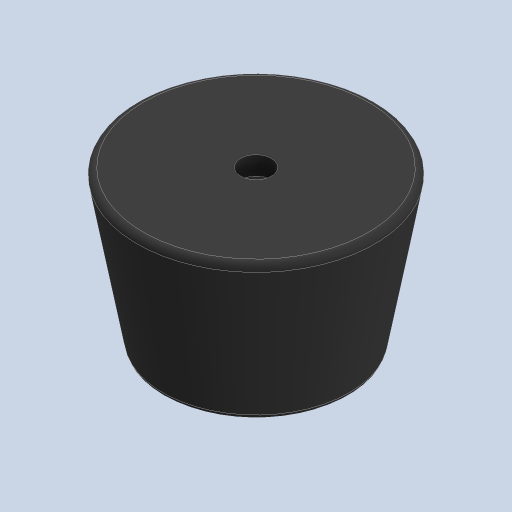
# Autodesk Inventor part: Pés
Saved by Autodesk Inventor 2023 (Build 270158000, 158)
## iProperties
Created: 2023-04-29
Part Number: Pés
Material: Rubber, Silicone
Document SubType Name: Sheet Metal
Designer: Mateus PC
Density: 1.25 g/cm^3
Sheet Metal Rule: Default_mm
Appearance: Rubber - Black
Mass: 12.8254 g
Surface Area: 66.7725 cm^2
Volume: 10.2603 cm^3
Author: Mateus PC
Autodesk Inventor part; units mm, degrees
ref_plane "YZ Plane" through (0, 0, 0) normal (1, 0, 0) x (0, 1, 0)
ref_plane "XZ Plane" through (0, 0, 0) normal (0, 1, 0) x (-1, 0, 0)
ref_plane "XY Plane" through (0, 0, 0) normal (0, 0, 1) x (1, 0, 0)
sketch "Sketch5" plane through (0, 0, 0) normal (0, 0, 1) x (1, 0, 0)
  line L0 (20, 0) -> (-20, 0) projected
  line L1 (-15.1481, 0.8228) -> (-19.2881, 23.8228)
  line L2 (-18.3039, 25) -> (-2.5, 25)
  line L3 (-2.5, 25) -> (-2.5, 22)
  line L4 (-2.5, 22) -> (-14.3283, 22)
  line L5 (-15.3159, 20.8429) -> (-12.1841, 1.1571)
  line L6 (-14.5, 0) -> (14.5, 0) projected
  arc A0 (-14.3283, 22) -> (-15.3159, 20.8429) centre (-14.3283, 21) ccw
  arc A1 (-18.3039, 25) -> (-19.2881, 23.8228) centre (-18.3039, 24) ccw
  line L7 (-14.1639, 0) -> (-13.1717, 0)
  arc A2 (-13.1717, 0) -> (-12.1841, 1.1571) centre (-13.1717, 1) ccw
  arc A3 (-15.1481, 0.8228) -> (-14.1639, 0) centre (-14.1639, 1) ccw
  line L8 (-28, 0) -> (28, 0) projected
  line L9 (0, -5.3193) -> (0, 30.3215) projected
  point P0 (0, 0)
  point P1 (-15, 0)
  point P2 (-19.5, 25)
  point P3 (-15.5, 22)
  point P4 (-12, 0)
  point P5 (0, 0)
  point P6 (0, 0)
  point P7 (-2.5, 23.5)
  dimension "d21" = 17
  dimension "d22" = 12
  dimension "d23" = 15
  dimension "d24" = 13
  dimension "d25" = 2.5
  dimension "d26" = 25
  dimension "d27" = 3
  dimension "d28" = 1
  dimension "d29" = 1
  constraints: 12 end point, 10 point on line, 8 point on circle, 8 tangent, 4 centre point, 3 midpoint, 2 equal radius, 2 perpendicular, 1 horizontal
  measures "d21" distance of point (-19.5, 25) L2.end
  measures "d22" distance of point (0, 0) point (-12, 0)
  measures "d23" distance of point (0, 0) point (-15, 0)
  measures "d24" distance of L3.end point (-15.5, 22)
  measures "d25" horizontal distance of point (0, 0) point (-2.5, 23.5)
  measures "d26" distance from line of point (0, 0) L2
  measures "d27" distance between parallel lines of L2 L4
  measures "d28" radius of A0
  measures "d29" radius of A2
revolve "Revolution1" add sketch "Sketch5" angle 360 about axis through (0, -10, 0) along (0, 1, 0)
equation "\"BendRadius\" = Thickness"
equation "\"BendReliefWidth\" = Thickness"
equation "\"BendReliefDepth\" = 0.5 * Thickness"
equation "\"CornerReliefSize\" = 4 * Thickness"
equation "\"MinimumRemnant\" = 2 * Thickness"
equation "\"TransitionRadius\" = BendRadius"
equation "\"JacobiRadiusSize\" = BendRadius"
equation "\"GapSize\" = Thickness"
equation "\"Thickness\" = 0.5"
body "Solid2"
